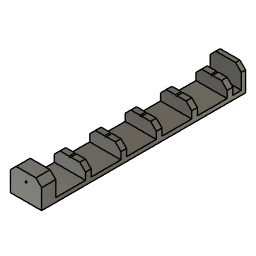
Led Connector Wire Jig (Autodesk Fusion 360 design; units mm, degrees)
Autodesk Fusion 360 part; units mm, degrees
sketch "Sketch1" plane through (0, 0, 0) normal (1, 0, 0) x (0, 1, 0)
  line L0 (0, 0) -> (10, 0)
  line L1 (10, 0) -> (10, -18)
  line L2 (10, -18) -> (0, -18)
  line L3 (0, -18) -> (0, 0)
  line L4 (0, -18) -> (35, -18)
  line L5 (35, -18) -> (35, -15)
  line L6 (35, -15) -> (0, -15)
  line L7 (0, -15) -> (0, -18)
  line L8 (35, -18) -> (31, -18)
  line L9 (31, -18) -> (31, -6)
  line L10 (31, -6) -> (35, -6)
  line L11 (35, -6) -> (35, -18)
  line L12 (10, 0) -> (31, 0)
  line L13 (31, 0) -> (31, -15)
  line L14 (31, -15) -> (10, -15)
  line L15 (10, -15) -> (10, 0)
  line L16 (35, 0) -> (56, 0)
  line L17 (60, -6) -> (60, -18)
  line L18 (56, -6) -> (60, -6)
  line L19 (56, 0) -> (56, -15)
  line L20 (56, -18) -> (56, -6)
  line L21 (60, -18) -> (56, -18)
  line L22 (25, -18) -> (60, -18)
  line L23 (60, -15) -> (25, -15)
  line L24 (35, -15) -> (35, 0)
  line L25 (35, 0) -> (35, -18)
  line L26 (60, 0) -> (81, 0)
  line L27 (85, -6) -> (85, -18)
  line L28 (81, -6) -> (85, -6)
  line L29 (81, 0) -> (81, -15)
  line L30 (81, -18) -> (81, -6)
  line L31 (85, -18) -> (81, -18)
  line L32 (50, -18) -> (85, -18)
  line L33 (85, -15) -> (50, -15)
  line L34 (60, -15) -> (60, 0)
  line L35 (60, 0) -> (60, -18)
  line L36 (85, 0) -> (106, 0)
  line L37 (110, -6) -> (110, -18)
  line L38 (106, -6) -> (110, -6)
  line L39 (106, 0) -> (106, -15)
  line L40 (106, -18) -> (106, -6)
  line L41 (110, -18) -> (106, -18)
  line L42 (75, -18) -> (110, -18)
  line L43 (110, -15) -> (75, -15)
  line L44 (85, -15) -> (85, 0)
  line L45 (85, 0) -> (85, -18)
  line L46 (110, 0) -> (131, 0)
  line L47 (135, -6) -> (135, -18)
  line L48 (131, -6) -> (135, -6)
  line L49 (131, 0) -> (131, -15)
  line L50 (131, -18) -> (131, -6)
  line L51 (135, -18) -> (131, -18)
  line L52 (100, -18) -> (135, -18)
  line L53 (135, -15) -> (100, -15)
  line L54 (110, -15) -> (110, 0)
  line L55 (110, 0) -> (110, -18)
  line L56 (135, -18) -> (141, -18)
  line L57 (141, -18) -> (141, -14.9934)
  line L58 (141, -14.9934) -> (135, -14.9934)
  line L59 (135, -14.9934) -> (135, -18)
  line L60 (141, -18) -> (144, -18)
  line L61 (144, -18) -> (144, 0)
  line L62 (144, 0) -> (141, 0)
  line L63 (141, 0) -> (141, -18)
  dimension "d1" = 10
  dimension "d2" = 18
  dimension "d3" = 35
  dimension "d4" = 3
  dimension "d5" = 4
  dimension "d6" = 12
  dimension "d17" = 21
  dimension "d20" = 100
  dimension "d21" = 0
  dimension "d22" = 6
  dimension "d23" = 3
  dimension "d24" = 18
  constraint horizontal L0
  constraint vertical L1
  constraint horizontal L2
  constraint vertical L3
  constraint coincident L0.start L3.end
  constraint horizontal L4
  constraint vertical L5
  constraint horizontal L6
  constraint vertical L7
  constraint horizontal L8
  constraint vertical L9
  constraint horizontal L10
  constraint vertical L11
  constraint horizontal L12
  constraint vertical L13
  constraint horizontal L14
  constraint vertical L15
  constraint coincident L6 L13.end
  constraint coincident L9 L13.end
  constraint horizontal L56
  constraint vertical L57
  constraint horizontal L58
  constraint vertical L59
  constraint horizontal L60
  constraint vertical L61
  constraint horizontal L62
  constraint vertical L63
  measures "d1" distance of L0.start L0.end
  measures "d2" distance of L0.start L2.end
  measures "d3" distance of L2.end L4.end
  measures "d4" distance of L2.end L6.end
  measures "d5" distance of L4.end L8.end
  measures "d6" distance of L4.end L10.end
  measures "d17" distance of L13.end L14.end
  measures "d22" distance of L47.end L56.end
  measures "d23" distance of L56.end L60.end
  measures "d24" distance of L56.end L62.end
extrude "Extrude1" add sketch "Sketch1" along normal blind 22 contours L0 L1 L3 L6 L15 | L1 L2 L3 L4 L6 L7 | L1 L4 L6 L9 L14 L22 L23 | L6 L9 L10 L11 L13 L23 L24 L25 | L4 L5 L6 L8 L9 L11 L22 L23 L25 | L5 L11 L20 L22 L23 L25 L32 L33 | L17 L20 L21 L22 L23 L32 L33 L35 | L17 L18 L19 L20 L23 L33 L34 L35 | L17 L30 L32 L33 L35 L42 L43 | L27 L30 L31 L32 L33 L42 L43 L45 | L27 L28 L29 L30 L33 L43 L44 L45 | L27 L40 L42 L43 L45 L52 L53 | L37 L40 L41 L42 L43 L52 L53 L55 | L37 L38 L39 L40 L43 L53 L54 L55 | L37 L50 L52 L53 L55 | L47 L50 L51 L52 L53 L59 | L47 L48 L49 L50 L53 L59 | L47 L56 L57 L58 L59 L63 | L57 L60 L61 L62 L63
sketch "Sketch2" plane through (0, 0, 0) normal (0, -1, 0) x (1, 0, 0)
  line L0 (0, 0) -> (0, -18)
  line L1 (0, -18) -> (22, -18)
  line L2 (22, -18) -> (22, 0)
  line L3 (22, 0) -> (0, 0)
  line L4 (0, 0) -> (22.1644, 0)
  line L5 (22.1644, 0) -> (22.1644, -6)
  line L6 (22.1644, -6) -> (0, -6)
  line L7 (0, -6) -> (0, 0)
  circle A0 centre (11.0822, -6) radius 0.5
  dimension "d9" = 6
  dimension "d10" = 1
  constraint horizontal L4
  constraint vertical L5
  constraint horizontal L6
  constraint vertical L7
  constraint coincident L0.start L3.end
  constraint midpoint L6 A0.centre
  measures "d9" distance of L0.start L6.end
  measures "d10" diameter of A0
hole "Hole1" at (11.0822, 0, -6) direction (0, 1, 0) diameter 1.2 depth 136 tip angle 140
chamfer "Chamfer1" distance 4 angle 45 14 edges at (0, 5, 0) (22, 5, 0) (0, 33, -6) (22, 33, -6) (22, 58, -6) (0, 58, -6) (0, 83, -6) (22, 83, -6) (0, 108, -6) (0, 133, -6) (22, 133, -6) (22, 108, -6) (22, 142.5, 0) (0, 142.5, 0)
